Autodesk Inventor part; units mm, degrees
(part 5 of 6)
sketch "Sketch63" plane through (-95.5889, -143.7847, 10) normal (0, 0, -1) x (-0.7071068, 0.7071068, 0)
  line L0 (0, 6) -> (1.7, 6) projected
  line L1 (0, 6) -> (0, 0) projected
  line L2 (0, 0) -> (1.7, 0) projected
  line L3 (1.7, 6) -> (1.7, 0) projected
  line L4 (10.7, 0) -> (10.7, 6) projected
  line L5 (10.7, 0) -> (12.4, 0) projected
  line L6 (12.4, 0) -> (12.4, 6) projected
  line L7 (10.7, 6) -> (12.4, 6) projected
  line L8 (3.058, 5.3026) -> (4.2659, 6) projected
  line L9 (4.2659, 6) -> (1.7, 6) projected
  line L10 (1.7, 0) -> (1.7, 6) projected
  line L11 (1.7, 0) -> (6.0424, 0) projected
  line L12 (6.0424, 0) -> (3.058, 1.723) projected
  line L13 (3.058, 1.723) -> (3.058, 5.3026) projected
  line L14 (8.0501, 6) -> (9.258, 5.3026) projected
  line L15 (9.258, 5.3026) -> (9.258, 1.723) projected
  line L16 (9.258, 1.723) -> (6.2736, 0) projected
  line L17 (6.2736, 0) -> (10.7, 0) projected
  line L18 (10.7, 6) -> (10.7, 0) projected
  line L19 (10.7, 6) -> (8.0501, 6) projected
  line L20 (4.2659, 6) -> (8.0501, 6) projected
  circle A0 centre (6.158, 3.5128) radius 1.5 projected
  line L21 (4.2659, 6) -> (8.0501, 6) projected
  line L22 (3.058, 5.3026) -> (4.2659, 6) projected
  line L23 (3.058, 1.723) -> (3.058, 5.3026) projected
  line L24 (6.0424, 0) -> (3.058, 1.723) projected
  line L25 (6.2736, 0) -> (6.0424, 0) projected
  line L26 (9.258, 1.723) -> (6.2736, 0) projected
  line L27 (9.258, 5.3026) -> (9.258, 1.723) projected
  line L28 (8.0501, 6) -> (9.258, 5.3026) projected
  line L29 (-79.2698, 64.6815) -> (-78.0677, 63.4794) projected
  line L30 (-79.2698, 64.6815) -> (-83.5124, 60.4388) projected
  line L31 (-83.5124, 60.4388) -> (-82.3103, 59.2367) projected
  line L32 (-78.0677, 63.4794) -> (-82.3103, 59.2367) projected
  line L33 (-77.6457, 61.952) -> (-76.1357, 61.5474) projected
  line L34 (-76.1357, 61.5474) -> (-78.0677, 63.4794) projected
  line L35 (-82.3103, 59.2367) -> (-78.0677, 63.4794) projected
  line L36 (-82.3103, 59.2367) -> (-79.3285, 56.2549) projected
  line L37 (-79.3285, 56.2549) -> (-80.1768, 59.4208) projected
  line L38 (-80.1768, 59.4208) -> (-77.6457, 61.952) projected
  circle A1 centre (-76.7192, 58.4944) radius 1.5 projected
  circle A2 centre (-76.7192, 58.4944) radius 1.5 projected
  line L39 (-76.1357, 61.5474) -> (-73.6662, 59.0779) projected
  line L40 (-77.6457, 61.952) -> (-76.1357, 61.5474) projected
  line L41 (-80.1768, 59.4208) -> (-77.6457, 61.952) projected
  line L42 (-79.3285, 56.2549) -> (-80.1768, 59.4208) projected
  line L43 (-78.9587, 55.8851) -> (-79.3285, 56.2549) projected
  line L44 (-75.7928, 55.0368) -> (-78.9587, 55.8851) projected
  line L45 (-73.2616, 57.5679) -> (-75.7928, 55.0368) projected
  line L46 (-73.6662, 59.0779) -> (-73.2616, 57.5679) projected
  line L47 (-75.9464, 52.8728) -> (-71.7037, 57.1154) projected
  line L48 (-73.6662, 59.0779) -> (-73.2616, 57.5679) projected
  line L49 (-73.2616, 57.5679) -> (-75.7928, 55.0368) projected
  line L50 (-75.7928, 55.0368) -> (-78.9587, 55.8851) projected
  line L51 (-78.9587, 55.8851) -> (-75.9464, 52.8728) projected
  line L52 (-71.7037, 57.1154) -> (-75.9464, 52.8728) projected
  line L53 (-71.7037, 57.1154) -> (-73.6662, 59.0779) projected
  line L54 (-75.9464, 52.8728) -> (-71.7037, 57.1154) projected
  line L55 (-75.9464, 52.8728) -> (-74.7443, 51.6707) projected
  line L56 (-74.7443, 51.6707) -> (-70.5017, 55.9133) projected
  line L57 (-71.7037, 57.1154) -> (-70.5017, 55.9133) projected
  line L58 (-101.1831, 147.5831) -> (-106.1831, 147.5831) projected
  line L59 (-106.1831, 135.1831) -> (-106.1831, 147.5831) projected
  line L60 (-106.1831, 135.1831) -> (-101.1831, 135.1831) projected
  line L61 (-101.1831, 135.1831) -> (-101.1831, 147.5831) projected
  circle A3 centre (-103.7792, 141.4107) radius 1.5 projected
  line L62 (-129.1831, 145.8831) -> (-135.1831, 145.8831) projected
  line L63 (-129.1831, 147.5831) -> (-135.1831, 147.5831) projected
  line L64 (-133.569, 144.5107) -> (-129.9894, 144.5107) projected
  line L65 (-135.1831, 141.7149) -> (-133.569, 144.5107) projected
  line L66 (-133.569, 144.5107) -> (-129.9894, 144.5107) projected
  line L67 (-129.9894, 144.5107) -> (-129.1831, 143.1142) projected
  line L68 (-129.1831, 143.1142) -> (-129.1831, 145.8831) projected
  line L69 (-135.1831, 145.8831) -> (-129.1831, 145.8831) projected
  line L70 (-135.1831, 145.8831) -> (-135.1831, 141.7149) projected
  line L71 (-129.1831, 147.5831) -> (-129.1831, 145.8831) projected
  line L72 (-129.1831, 147.5831) -> (-135.1831, 147.5831) projected
  line L73 (-135.1831, 147.5831) -> (-135.1831, 145.8831) projected
  line L74 (-129.1831, 145.8831) -> (-135.1831, 145.8831) projected
  circle A4 centre (-131.7792, 141.4107) radius 1.5 projected
  line L75 (-135.1831, 141.1065) -> (-135.1831, 141.7149) projected
  line L76 (-133.569, 138.3107) -> (-135.1831, 141.1065) projected
  line L77 (-129.9894, 138.3107) -> (-133.569, 138.3107) projected
  line L78 (-129.1831, 139.7072) -> (-129.9894, 138.3107) projected
  line L79 (-129.1831, 143.1142) -> (-129.1831, 139.7072) projected
  line L80 (-129.9894, 144.5107) -> (-129.1831, 143.1142) projected
  line L81 (-133.569, 144.5107) -> (-129.9894, 144.5107) projected
  line L82 (-135.1831, 141.7149) -> (-133.569, 144.5107) projected
  line L83 (-133.569, 138.3107) -> (-135.1831, 141.1065) projected
  line L84 (-135.1831, 141.1065) -> (-135.1831, 136.8831) projected
  line L85 (-129.1831, 136.8831) -> (-135.1831, 136.8831) projected
  line L86 (-129.1831, 136.8831) -> (-129.1831, 139.7072) projected
  line L87 (-129.1831, 139.7072) -> (-129.9894, 138.3107) projected
  line L88 (-129.9894, 138.3107) -> (-133.569, 138.3107) projected
  line L89 (-135.1831, 135.1831) -> (-129.1831, 135.1831) projected
  line L90 (-135.1831, 136.8831) -> (-129.1831, 136.8831) projected
  line L91 (-135.1831, 136.8831) -> (-135.1831, 135.1831) projected
  line L92 (-135.1831, 135.1831) -> (-129.1831, 135.1831) projected
  line L93 (-129.1831, 136.8831) -> (-129.1831, 135.1831) projected
  line L94 (-79.6081, 145.9581) -> (-79.6081, 136.8081) projected
  line L95 (-86.1831, 145.9581) -> (-79.6081, 145.9581) projected
  line L96 (-86.1831, 136.8081) -> (-86.1831, 145.9581) projected
  line L97 (-86.1831, 136.8081) -> (-79.6081, 136.8081) projected
  line L98 (-86.1831, 145.9581) -> (-79.6081, 145.9581) projected
  line L99 (-79.6081, 145.9581) -> (-79.6081, 147.9581) projected
  line L100 (-79.6081, 147.9581) -> (-86.1831, 147.9581) projected
  line L101 (-86.1831, 147.9581) -> (-86.1831, 145.9581) projected
  line L102 (-86.1831, 136.8081) -> (-79.6081, 136.8081) projected
  line L103 (-86.1831, 136.8081) -> (-86.1831, 134.8081) projected
  line L104 (-86.1831, 134.8081) -> (-79.6081, 134.8081) projected
  line L105 (-79.6081, 134.8081) -> (-79.6081, 136.8081) projected
  line L106 (-43.4494, 188.6918) -> (-43.4494, 182.1168) projected
  line L107 (-43.4494, 188.6918) -> (-45.4494, 188.6918) projected
  line L108 (-45.4494, 188.6918) -> (-45.4494, 182.1168) projected
  line L109 (-45.4494, 182.1168) -> (-43.4494, 182.1168) projected
  line L110 (-34.2994, 182.1168) -> (-43.4494, 182.1168) projected
  line L111 (-34.2994, 188.6918) -> (-34.2994, 182.1168) projected
  line L112 (-43.4494, 188.6918) -> (-34.2994, 188.6918) projected
  line L113 (-43.4494, 188.6918) -> (-43.4494, 182.1168) projected
  line L114 (-34.2994, 188.6918) -> (-34.2994, 182.1168) projected
  line L115 (-34.2994, 182.1168) -> (-32.2994, 182.1168) projected
  line L116 (-32.2994, 182.1168) -> (-32.2994, 188.6918) projected
  line L117 (-32.2994, 188.6918) -> (-34.2994, 188.6918) projected
  circle A5 centre (-38.9335, 206.21) radius 1.5 projected
  line L118 (-32.6744, 203.6918) -> (-32.6744, 208.6918) projected
  line L119 (-45.0744, 208.6918) -> (-32.6744, 208.6918) projected
  line L120 (-45.0744, 208.6918) -> (-45.0744, 203.6918) projected
  line L121 (-45.0744, 203.6918) -> (-32.6744, 203.6918) projected
  line L122 (-35.8335, 232.4202) -> (-37.0951, 231.6918) projected
  line L123 (-37.0951, 231.6918) -> (-34.3744, 231.6918) projected
  line L124 (-34.3744, 237.6918) -> (-34.3744, 231.6918) projected
  line L125 (-34.3744, 237.6918) -> (-38.7642, 237.6918) projected
  line L126 (-38.7642, 237.6918) -> (-35.8335, 235.9998) projected
  line L127 (-35.8335, 235.9998) -> (-35.8335, 232.4202) projected
  line L128 (-32.6744, 231.6918) -> (-34.3744, 231.6918) projected
  line L129 (-32.6744, 231.6918) -> (-32.6744, 237.6918) projected
  line L130 (-32.6744, 237.6918) -> (-34.3744, 237.6918) projected
  line L131 (-34.3744, 231.6918) -> (-34.3744, 237.6918) projected
  circle A6 centre (-38.9335, 234.21) radius 1.5 projected
  line L132 (-37.0951, 231.6918) -> (-40.7719, 231.6918) projected
  line L133 (-35.8335, 232.4202) -> (-37.0951, 231.6918) projected
  line L134 (-35.8335, 235.9998) -> (-35.8335, 232.4202) projected
  line L135 (-38.7642, 237.6918) -> (-35.8335, 235.9998) projected
  line L136 (-39.1028, 237.6918) -> (-38.7642, 237.6918) projected
  line L137 (-42.0335, 235.9998) -> (-39.1028, 237.6918) projected
  line L138 (-42.0335, 232.4202) -> (-42.0335, 235.9998) projected
  line L139 (-40.7719, 231.6918) -> (-42.0335, 232.4202) projected
  line L140 (-42.0335, 235.9998) -> (-39.1028, 237.6918) projected
  line L141 (-43.3744, 237.6918) -> (-43.3744, 231.6918) projected
  line L142 (-43.3744, 237.6918) -> (-43.3744, 231.6918) projected
  line L143 (-43.3744, 237.6918) -> (-45.0744, 237.6918) projected
  line L144 (-45.0744, 237.6918) -> (-45.0744, 231.6918) projected
  line L145 (-43.3744, 231.6918) -> (-45.0744, 231.6918) projected
  line L146 (-40.7719, 231.6918) -> (-42.0335, 232.4202) projected
  line L147 (-42.0335, 232.4202) -> (-42.0335, 235.9998) projected
  line L148 (-42.0335, 235.9998) -> (-39.1028, 237.6918) projected
  line L149 (-39.1028, 237.6918) -> (-43.3744, 237.6918) projected
  line L150 (-43.3744, 231.6918) -> (-43.3744, 237.6918) projected
  line L151 (-43.3744, 231.6918) -> (-40.7719, 231.6918) projected
  line L152 (3.9214, 145.5746) -> (8.5707, 150.2238) projected
  line L153 (3.9214, 145.5746) -> (8.5707, 150.2238) projected
  line L154 (8.5707, 150.2238) -> (7.1565, 151.638) projected
  line L155 (7.1565, 151.638) -> (2.5072, 146.9888) projected
  line L156 (2.5072, 146.9888) -> (3.9214, 145.5746) projected
  line L157 (10.3915, 139.1046) -> (3.9214, 145.5746) projected
  line L158 (10.3915, 139.1046) -> (15.0407, 143.7538) projected
  line L159 (8.5707, 150.2238) -> (15.0407, 143.7538) projected
  line L160 (3.9214, 145.5746) -> (8.5707, 150.2238) projected
  line L161 (10.3915, 139.1046) -> (15.0407, 143.7538) projected
  line L162 (10.3915, 139.1046) -> (11.8057, 137.6904) projected
  line L163 (11.8057, 137.6904) -> (16.4549, 142.3396) projected
  line L164 (16.4549, 142.3396) -> (15.0407, 143.7538) projected
  line L165 (26.7963, 153.2113) -> (30.3319, 156.7469) projected
  line L166 (21.5638, 165.515) -> (30.3319, 156.7469) projected
  line L167 (21.5638, 165.515) -> (18.0282, 161.9795) projected
  line L168 (18.0282, 161.9795) -> (26.7963, 153.2113) projected
  circle A7 centre (24.1798, 159.3656) radius 1.5 projected
  line L169 (43.2719, 184.819) -> (39.0293, 180.5764) projected
  line L170 (43.2719, 184.819) -> (42.0699, 186.0211) projected
  line L171 (42.0699, 186.0211) -> (37.8272, 181.7785) projected
  line L172 (39.0293, 180.5764) -> (37.8272, 181.7785) projected
  line L173 (40.8896, 178.7161) -> (40.5212, 180.0911) projected
  line L174 (40.5212, 180.0911) -> (43.0523, 182.6222) projected
  line L175 (43.0523, 182.6222) -> (46.3532, 181.7377) projected
  line L176 (46.3532, 181.7377) -> (43.2719, 184.819) projected
  line L177 (39.0293, 180.5764) -> (43.2719, 184.819) projected
  line L178 (39.0293, 180.5764) -> (40.8896, 178.7161) projected
  circle A8 centre (43.9788, 179.1646) radius 1.5 projected
  line L179 (43.5302, 176.0754) -> (40.8896, 178.7161) projected
  line L180 (44.9052, 175.707) -> (43.5302, 176.0754) projected
  line L181 (47.4364, 178.2381) -> (44.9052, 175.707) projected
  line L182 (46.5519, 181.5391) -> (47.4364, 178.2381) projected
  line L183 (46.3532, 181.7377) -> (46.5519, 181.5391) projected
  line L184 (43.0523, 182.6222) -> (46.3532, 181.7377) projected
  line L185 (40.5212, 180.0911) -> (43.0523, 182.6222) projected
  line L186 (40.8896, 178.7161) -> (40.5212, 180.0911) projected
  line L187 (44.9052, 175.707) -> (43.5302, 176.0754) projected
  line L188 (43.5302, 176.0754) -> (45.3933, 174.2124) projected
  line L189 (49.6359, 178.4551) -> (45.3933, 174.2124) projected
  line L190 (49.6359, 178.4551) -> (46.5519, 181.5391) projected
  line L191 (46.5519, 181.5391) -> (47.4364, 178.2381) projected
  line L192 (47.4364, 178.2381) -> (44.9052, 175.707) projected
  line L193 (46.5953, 173.0103) -> (45.3933, 174.2124) projected
  line L194 (46.5953, 173.0103) -> (50.838, 177.253) projected
  line L195 (50.838, 177.253) -> (49.6359, 178.4551) projected
  line L196 (45.3933, 174.2124) -> (49.6359, 178.4551) projected
  line L197 (46.9337, 91.7337) -> (46.9337, 100.8837) projected
  line L198 (53.5087, 91.7337) -> (46.9337, 91.7337) projected
  line L199 (53.5087, 100.8837) -> (53.5087, 91.7337) projected
  line L200 (53.5087, 100.8837) -> (46.9337, 100.8837) projected
  line L201 (53.5087, 100.8837) -> (46.9337, 100.8837) projected
  line L202 (53.5087, 100.8837) -> (53.5087, 102.8837) projected
  line L203 (53.5087, 102.8837) -> (46.9337, 102.8837) projected
  line L204 (46.9337, 102.8837) -> (46.9337, 100.8837) projected
  line L205 (53.5087, 91.7337) -> (46.9337, 91.7337) projected
  line L206 (46.9337, 91.7337) -> (46.9337, 89.7337) projected
  line L207 (46.9337, 89.7337) -> (53.5087, 89.7337) projected
  line L208 (53.5087, 89.7337) -> (53.5087, 91.7337) projected
  circle A9 centre (71.0354, 96.2907) radius 1.5 projected
  line L209 (68.5087, 90.1087) -> (73.5087, 90.1087) projected
  line L210 (73.5087, 102.5087) -> (73.5087, 90.1087) projected
  line L211 (73.5087, 102.5087) -> (68.5087, 102.5087) projected
  line L212 (68.5087, 102.5087) -> (68.5087, 90.1087) projected
  line L213 (102.5087, 100.8087) -> (96.5087, 100.8087) projected
  line L214 (102.5087, 100.8087) -> (102.5087, 102.5087) projected
  line L215 (102.5087, 102.5087) -> (96.5087, 102.5087) projected
  line L216 (96.5087, 100.8087) -> (96.5087, 102.5087) projected
  line L217 (100.8251, 99.3907) -> (102.5087, 96.4747) projected
  line L218 (102.5087, 96.4747) -> (102.5087, 100.8087) projected
  line L219 (96.5087, 100.8087) -> (102.5087, 100.8087) projected
  line L220 (96.5087, 100.8087) -> (96.5087, 98.1143) projected
  line L221 (96.5087, 98.1143) -> (97.2456, 99.3907) projected
  line L222 (97.2456, 99.3907) -> (100.8251, 99.3907) projected
  circle A10 centre (99.0354, 96.2907) radius 1.5 projected
  line L223 (102.5087, 96.4747) -> (102.5087, 96.1066) projected
  line L224 (100.8251, 99.3907) -> (102.5087, 96.4747) projected
  line L225 (97.2456, 99.3907) -> (100.8251, 99.3907) projected
  line L226 (96.5087, 98.1143) -> (97.2456, 99.3907) projected
  line L227 (96.5087, 94.467) -> (96.5087, 98.1143) projected
  line L228 (97.2456, 93.1907) -> (96.5087, 94.467) projected
  line L229 (100.8251, 93.1907) -> (97.2456, 93.1907) projected
  line L230 (102.5087, 96.1066) -> (100.8251, 93.1907) projected
  line L231 (102.5087, 96.1066) -> (100.8251, 93.1907) projected
  line L232 (100.8251, 93.1907) -> (97.2456, 93.1907) projected
  line L233 (97.2456, 93.1907) -> (96.5087, 94.467) projected
  line L234 (96.5087, 94.467) -> (96.5087, 91.8087) projected
  line L235 (102.5087, 91.8087) -> (96.5087, 91.8087) projected
  line L236 (102.5087, 91.8087) -> (102.5087, 96.1066) projected
  line L237 (96.5087, 90.1087) -> (96.5087, 91.8087) projected
  line L238 (96.5087, 90.1087) -> (102.5087, 90.1087) projected
  line L239 (102.5087, 90.1087) -> (102.5087, 91.8087) projected
  line L240 (96.5087, 91.8087) -> (102.5087, 91.8087) projected
  circle A11 centre (6.158, 31.5128) radius 1.5 projected
  line L241 (0, 34) -> (0, 29) projected
  line L242 (12.4, 29) -> (0, 29) projected
  line L243 (12.4, 29) -> (12.4, 34) projected
  line L244 (12.4, 34) -> (0, 34) projected
  line L245 (1.625, 55.575) -> (10.775, 55.575) projected
  line L246 (1.625, 49) -> (1.625, 55.575) projected
  line L247 (10.775, 49) -> (1.625, 49) projected
  line L248 (10.775, 49) -> (10.775, 55.575) projected
  line L249 (1.625, 49) -> (1.625, 55.575) projected
  line L250 (1.625, 55.575) -> (-0.375, 55.575) projected
  line L251 (-0.375, 55.575) -> (-0.375, 49) projected
  line L252 (-0.375, 49) -> (1.625, 49) projected
  line L253 (10.775, 49) -> (10.775, 55.575) projected
  line L254 (10.775, 49) -> (12.775, 49) projected
  line L255 (12.775, 49) -> (12.775, 55.575) projected
  line L256 (12.775, 55.575) -> (10.775, 55.575) projected
  line L257 (-47.7151, 93.938) -> (-43.0659, 98.5872) projected
  line L258 (-43.0659, 98.5872) -> (-44.4801, 100.0015) projected
  line L259 (-44.4801, 100.0015) -> (-49.1294, 95.3522) projected
  line L260 (-49.1294, 95.3522) -> (-47.7151, 93.938) projected
  line L261 (-43.0659, 98.5872) -> (-36.5959, 92.1172) projected
  line L262 (-47.7151, 93.938) -> (-43.0659, 98.5872) projected
  line L263 (-41.2451, 87.468) -> (-47.7151, 93.938) projected
  line L264 (-41.2451, 87.468) -> (-36.5959, 92.1172) projected
  line L265 (-41.2451, 87.468) -> (-36.5959, 92.1172) projected
  line L266 (-41.2451, 87.468) -> (-39.8309, 86.0538) projected
  line L267 (-39.8309, 86.0538) -> (-35.1817, 90.703) projected
  line L268 (-35.1817, 90.703) -> (-36.5959, 92.1172) projected
  line L269 (-59.4708, 84.4805) -> (-63.0063, 80.9449) projected
  line L270 (-54.2382, 72.1768) -> (-63.0063, 80.9449) projected
  line L271 (-54.2382, 72.1768) -> (-50.7027, 75.7123) projected
  line L272 (-50.7027, 75.7123) -> (-59.4708, 84.4805) projected
  circle A12 centre (-56.9202, 78.2934) radius 1.5 projected
  point P0 (34.0795, 169.2627)
  point P1 (-75.9464, 52.8728)
  point P2 (-71.7037, 57.1154)
  point P3 (-73.6662, 59.0779)
  point P4 (-76.1357, 61.5474)
  point P5 (-78.0677, 63.4794)
  point P6 (96.5087, 94.467)
  point P7 (96.5087, 91.8087)
  point P8 (102.5087, 91.8087)
  point P9 (102.5087, 96.1066)
  point P10 (102.5087, 96.4747)
  point P11 (46.9337, 100.8837)
  point P12 (46.9337, 91.7337)
  point P13 (53.5087, 91.7337)
  point P14 (53.5087, 100.8837)
  point P15 (15.0407, 143.7538)
  point P16 (8.5707, 150.2238)
  point P17 (3.9214, 145.5746)
  point P18 (10.3915, 139.1046)
  point P19 (46.3532, 181.7377)
  point P20 (43.2719, 184.819)
  point P21 (39.0293, 180.5764)
  point P22 (40.8896, 178.7161)
  point P23 (43.5302, 176.0754)
  point P24 (45.3933, 174.2124)
  point P25 (49.6359, 178.4551)
  point P26 (46.5519, 181.5391)
  point P27 (-43.4494, 182.1168)
  point P28 (-34.2994, 182.1168)
  point P29 (-34.2994, 188.6918)
  point P30 (-43.4494, 188.6918)
  point P31 (-43.3744, 237.6918)
  point P32 (-40.7719, 231.6918)
  point P33 (-37.0951, 231.6918)
  point P34 (-34.3744, 231.6918)
  point P35 (-34.3744, 237.6918)
  point P36 (-38.7642, 237.6918)
  point P37 (-39.1028, 237.6918)
  point P38 (-135.1831, 145.8831)
  point P39 (-135.1831, 141.7149)
  point P40 (-135.1831, 141.1065)
  point P41 (-129.1831, 143.1142)
  point P42 (-129.1831, 145.8831)
  point P43 (-129.1831, 147.5831)
  point P44 (-79.6081, 136.8081)
  point P45 (-79.6081, 145.9581)
  point P46 (-86.1831, 145.9581)
  point P47 (-86.1831, 136.8081)
  point P48 (-47.7151, 93.938)
  point P49 (-41.2451, 87.468)
  point P50 (-43.0659, 98.5872)
  point P51 (1.625, 49)
  point P52 (10.775, 49)
  point P53 (10.775, 55.575)
  point P54 (1.625, 55.575)
  point P55 (10.7, 6)
  point P56 (1.7, 0)
  point P57 (6.0424, 0)
  point P58 (6.2736, 0)
  point P59 (10.7, 0)
extrude "Extrusion60" cut sketch "Sketch63" against normal blind 19 contours L0 L3 L2 L1 | L9 L8 L13 L12 L11 L3 | L20 L14 L15 L16 L25 L12 L13 L8 | L19 L4 L17 L16 L15 L14 | L7 L6 L5 L4 | L29 L32 L31 L30 | L34 L33 L38 L37 L36 L32 | L39 L46 L45 L44 L43 L37 L38 L33 | L53 L47 L51 L44 L45 L46 | L57 L56 L55 L47 | A1 | L61 L60 L59 L58 | L68 L67 L64 L65 L70 L62 | L62 L73 L63 L71 | L79 L78 L77 L76 L75 L65 L64 L67 | L86 L85 L84 L76 L77 L78 | L93 L89 L91 L85 | A4 | L94 L97 L96 L95 | L95 L101 L100 L99 | L105 L104 L103 L97 | L112 L111 L110 L106 | L106 L109 L108 L107 | L117 L116 L115 L111 | L121 L120 L119 L118 | L127 L126 L125 L124 L123 L122 | L122 L132 L139 L138 L137 L136 L126 L127 | L124 L130 L129 L128 | L151 L141 L149 L137 L138 L139 | L145 L144 L143 L141 | L156 L155 L154 L152 | L152 L159 L158 L157 | L158 L164 L163 L162 | L168 L167 L166 L165 | L176 L175 L174 L173 L178 L169 | L169 L172 L171 L170 | L183 L182 L181 L180 L179 L173 L174 L175 | L190 L189 L188 L180 L181 L182 | L195 L194 L193 L189 | A8 | L197 L200 L199 L198 | L198 L208 L207 L206 | L204 L203 L202 L200 | A9 | L212 L211 L210 L209 | L218 L217 L222 L221 L220 L213 | L213 L216 L215 L214 | L223 L230 L229 L228 L227 L221 L222 L217 | L236 L235 L234 L228 L229 L230 | L239 L238 L237 L235 | A10 | L244 L243 L242 L241 | L245 L248 L247 L246 | L246 L252 L251 L250 | L256 L255 L254 L248 | L260 L259 L258 L257 | L257 L261 L264 L263 | L264 L268 L267 L266 | L272 L271 L270 L269
sketch "Sketch66" plane through (9.4148, -138.9501, 55) normal (0, 0, -1) x (-1, 0, 0)
  line L0 (-45.5215, 41.2849) -> (-35.0215, 41.2849)
  line L1 (-31.4215, 41.2849) -> (-20.9215, 41.2849)
  line L2 (-17.3215, 41.2849) -> (-6.8215, 41.2849)
  line L3 (-3.2285, 41.2849) -> (31.7715, 41.2849)
  line L4 (-74.8673, 64.1) -> (-74.8673, 71.1) projected
  line L5 (77.0633, 52.65) -> (77.0633, 82.65) projected
  arc A0 (-40.1627, 65.6758) -> (-45.5215, 41.2849) centre (7.9948, 42.3113) ccw
  arc A1 (-28.0472, 65.6798) -> (-35.0215, 41.2849) centre (4.8127, 43.091) ccw
  arc A2 (-23.5743, 65.6813) -> (-31.4215, 41.2849) centre (4.8107, 43.0909) ccw
  arc A3 (-7.8955, 65.6864) -> (-20.9215, 41.2849) centre (5.751, 42.7242) ccw
  arc A4 (2.9932, 65.69) -> (-17.3215, 41.2849) centre (5.416, 43.0158) ccw
  arc A5 (4.8107, 55.3031) -> (-6.8215, 41.2849) centre (5.3934, 42.9843) ccw
  arc A6 (4.8107, 51.7737) -> (-3.2285, 41.2849) centre (5.7806, 42.7051) ccw
  arc A7 (-39.2025, 67.5594) -> (-40.1627, 65.6758) centre (7.9948, 42.3113) ccw
  arc A8 (-45.5215, 94.0365) -> (-39.2025, 67.5594) centre (6.2562, 92.4012) ccw
  line L6 (-45.5215, 94.0365) -> (-35.0215, 94.0365)
  line L7 (-31.4215, 94.0365) -> (-20.9215, 94.0365)
  line L8 (-17.3215, 94.0365) -> (-6.8215, 94.0365)
  line L9 (-3.2215, 94.0365) -> (31.7785, 94.0365)
  arc A9 (31.7715, 41.2849) -> (31.7785, 94.0365) centre (30.1154, 67.6609) ccw
  arc A10 (-26.5935, 67.6609) -> (-28.0472, 65.6798) centre (4.8127, 43.091) ccw
  arc A11 (-35.0215, 94.0365) -> (-26.5935, 67.6609) centre (5.544, 92.4644) ccw
  arc A12 (-21.8792, 67.6609) -> (-23.5743, 65.6813) centre (4.8107, 43.0909) ccw
  arc A13 (-31.4215, 94.0365) -> (-21.8792, 67.6609) centre (3.6645, 91.8162) ccw
  arc A14 (-4.0829, 67.5594) -> (-7.8955, 65.6864) centre (5.751, 42.7242) ccw
  arc A15 (-20.9215, 94.0365) -> (-4.0829, 67.5594) centre (5.8906, 92.4952) ccw
  line L10 (4.8107, 51.7737) -> (30.8107, 51.7737)
  line L11 (4.8107, 55.3031) -> (30.8107, 55.3031)
  line L12 (4.8107, 79.8559) -> (30.8107, 79.8559)
  arc A16 (-6.8215, 94.0365) -> (4.8107, 79.8559) centre (5.796, 92.5253) ccw
  arc A17 (30.8107, 55.3031) -> (42.559, 65.703) centre (29.9904, 68.0655) ccw
  line L13 (2.9932, 65.69) -> (42.559, 65.703)
  line L14 (2.9932, 69.2913) -> (42.5593, 69.2913)
  arc A18 (42.5593, 69.2913) -> (30.8107, 79.8559) centre (29.7982, 66.9149) ccw
  arc A19 (-17.3215, 94.0365) -> (2.9932, 69.2913) centre (6.0846, 92.5405) ccw
  line L15 (30.8622, 83.4409) -> (4.8622, 83.4409)
  arc A20 (-3.2215, 94.0365) -> (4.8622, 83.4409) centre (6.2101, 92.8507) ccw
  arc A21 (30.8107, 51.7737) -> (30.8622, 83.4409) centre (30.389, 67.608) ccw
  line L16 (-30.6501, 104.1104) -> (-26.9242, 104.1104) projected
  line L17 (-26.9242, 31.1897) -> (-30.6501, 31.1897) projected
  line L18 (0, 0) -> (18.8297, 0) projected
  line L19 (0, 135.3001) -> (0, 134.0127) projected
  point P0 (9.4148, 138.9501)
  point P1 (-23.5743, 65.6813)
  dimension "d833" = 10.5
  dimension "d834" = 10.5
  dimension "d835" = 3.6
  dimension "d836" = 10.5
  dimension "d837" = 3.6
  dimension "d838" = 35
  dimension "d839" = 3.593
  dimension "d842" = 10.5
  dimension "d843" = 10.5
  dimension "d844" = 3.6
  dimension "d845" = 10.5
  dimension "d846" = 3.6
  dimension "d847" = 35
  dimension "d848" = 3.6
  dimension "d849" = 26
  dimension "d850" = 26
  dimension "d851" = 26
  dimension "d882" = 34.504
  dimension "d883" = 34.5043
  dimension "d884" = 45.2848
  dimension "d886" = 46.2526
  dimension "d896" = 72.2506
  dimension "d900" = 81.1462
  dimension "d901" = 98.9425
  dimension "d902" = 26
  dimension "d905" = 14.1496
  dimension "d911" = 10.0952
  dimension "d912" = 10.0739
  dimension "d913" = 15.8399
  dimension "d914" = 26.428
  dimension "d915" = 12.7888
  dimension "d916" = 12.9805
  dimension "d917" = 53.5261
  dimension "d918" = 51.8036
  dimension "d919" = 9.5059
  dimension "d920" = 23.4538
  dimension "d921" = 26.8564
  dimension "d922" = 12.7077
  dimension "d923" = 9.1203
  dimension "d924" = 26.7113
  dimension "d925" = 26.7113
  dimension "d926" = 40.5959
  dimension "d927" = 22.8033
  dimension "d928" = 12.3325
  dimension "d929" = 39.8752
  dimension "d930" = 39.8752
  dimension "d931" = 36.2772
  dimension "d932" = 36.2772
  dimension "d933" = 35.1562
  dimension "d934" = 89.981
  dimension "d935" = 69.2913
  dimension "d936" = 55.303
  dimension "d937" = 51.7737
  dimension "d938" = 79.8559
  dimension "d939" = 41.2849
  dimension "d940" = 94.0365
  dimension "d941" = 41.2849
  dimension "d942" = 94.0365
  dimension "d943" = 41.2849
  dimension "d944" = 16.9356
  dimension "d945" = 45.2918
  dimension "d946" = 46.2011
  dimension "d947" = 69.0685
  dimension "d948" = 70.8071
  constraints: 46 point on circle, 28 end point, 22 centre point, 13 horizontal, 2 vertical alignment, 1 concentric, 1 point on line
  measures "d833" distance of L0.start L0.end
  measures "d834" distance of L1.start L1.end
  measures "d835" distance of L1.start L0.end
  measures "d836" distance of L2.start L2.end
  measures "d837" distance of L2.start L1.end
  measures "d838" distance of L3.start L3.end
  measures "d839" distance of L3.start L2.end
  measures "d842" distance of L6.start L6.end
  measures "d843" distance of L7.start L7.end
  measures "d844" distance of L7.start L6.end
  measures "d845" distance of L8.start L8.end
  measures "d846" distance of L8.start L7.end
  measures "d847" distance of L9.start L9.end
  measures "d848" distance of L9.start L8.end
  measures "d849" distance of L10.start L10.end
  measures "d850" distance of L11.start L11.end
  measures "d851" distance of L12.start L12.end
  measures "d882" distance from line of L14.end L5
  measures "d883" distance from line of L13.end L5
  measures "d884" distance from line of L9.end L5
  measures "d886" distance from line of L12.end L5
  measures "d896" distance from line of A10.centre L5
  measures "d900" distance from line of A14.start L5
  measures "d901" distance from line of A12.start L5
  measures "d902" distance of L15.start L15.end
  measures "d905" distance between parallel lines of L15 L14
  measures "d911" distance between parallel lines of L1 L17
  measures "d912" distance between parallel lines of L16 L7
  measures "d913" radius of A21
  measures "d914" radius of A9
  measures "d915" radius of A17
  measures "d916" radius of A18
  measures "d917" radius of A0
  measures "d918" radius of A8
  measures "d919" radius of A20
  measures "d920" radius of A19
  measures "d921" radius of A15
  measures "d922" radius of A16
  measures "d923" radius of A6
  measures "d924" radius of A3
  measures "d925" radius of A14
  measures "d926" radius of A11
  measures "d927" radius of A4
  measures "d928" radius of A5
  measures "d929" radius of A1
  measures "d930" radius of A10
  measures "d931" radius of A2
  measures "d932" radius of A12
  measures "d933" radius of A13
  measures "d934" angle of L19 L13
  measures "d935" distance between parallel lines of L18 L14
  measures "d936" distance between parallel lines of L18 L11
  measures "d937" distance between parallel lines of L18 L10
  measures "d938" distance between parallel lines of L18 L12
  measures "d939" distance between parallel lines of L18 L3
  measures "d940" distance between parallel lines of L18 L9
  measures "d941" distance between parallel lines of L18 L2
  measures "d942" distance between parallel lines of L18 L6
  measures "d943" distance between parallel lines of L18 L0
  measures "d944" distance from line of L5.end L13
  measures "d945" distance from line of L3.end L5
  measures "d946" distance from line of L15.start L5
  measures "d947" distance from line of A0.centre L5
  measures "d948" distance from line of A8.centre L5
extrude "Extrusion61" cut sketch "Sketch66" against normal blind 92.5
sketch "Sketch67" plane through (88.2822, -48.8001, 10) normal (1, 0, 0) x (0, 0, -1)
  line L0 (0, -22.5) -> (-58.1963, -22.5) projected
  line L1 (0, -45) -> (0, 0) projected
  line L2 (-56.7845, 0) -> (0, 0) projected
  line L3 (0, -45) -> (-56.7845, -45) projected
  line L4 (-6.15, -26.05) -> (-6.15, -19.05) projected
  arc A0 (-2.35, -19.05) -> (-6.15, -19.05) centre (-4.25, -19.05) ccw projected
  line L5 (-2.35, -19.05) -> (-2.35, -26.05) projected
  arc A1 (-6.15, -26.05) -> (-2.35, -26.05) centre (-4.25, -26.05) ccw projected
  circle A2 centre (-3.5, -1.55) radius 1 projected
  circle A3 centre (-12, -9.05) radius 8.15 projected
  circle A4 centre (-20.5, -1.55) radius 1 projected
  circle A5 centre (-20.5, -43.55) radius 1 projected
  circle A6 centre (-12, -36.05) radius 8.15 projected
  circle A7 centre (-3.5, -43.55) radius 1 projected
  line L6 (0, -45) -> (-25, -45)
  line L7 (-25, -45) -> (-25, 0)
  line L8 (-25, 0) -> (0, 0)
  line L9 (0, 0) -> (0, -45)
  arc A8 (-56.7845, 0) -> (-56.7845, -45) centre (121.8037, -22.5) ccw projected
  point P0 (10, 48.8001)
  dimension "d966" = 25
  constraints: 8 end point, 2 parallel, 1 horizontal, 1 perpendicular, 1 point on line
  measures "d966" distance of L7.end L8.end
extrude "Extrusion62" cut sketch "Sketch67" against normal blind 10 contours L1 L3 L7 L0 L4 A1 L5 | L0 L5 A0 L4 L7 L2 L1 | L5 A1 L4 L0 | L0 L4 A0 L5 | A2 | A3 | A4 | A5 | A6 | A7
sketch "Sketch71" plane through (9.4148, -138.9501, 55) normal (0, 0, -1) x (-1, 0, 0)
  line L0 (2.9932, 65.69) -> (42.559, 65.703) projected
  arc A0 (30.8107, 55.3031) -> (42.559, 65.703) centre (29.9904, 68.0655) ccw projected
  line L1 (30.8107, 55.3031) -> (4.8107, 55.3031) projected
  arc A1 (4.8107, 55.3031) -> (-6.8215, 41.2849) centre (5.3934, 42.9843) ccw projected
  line L2 (-6.8215, 41.2849) -> (-17.3215, 41.2849) projected
  arc A2 (2.9932, 65.69) -> (-17.3215, 41.2849) centre (5.416, 43.0158) ccw projected
  arc A3 (-20.9215, 94.0365) -> (-4.0829, 67.5594) centre (5.8906, 92.4952) ccw projected
  arc A4 (-4.0829, 67.5594) -> (-20.9215, 41.2849) centre (5.751, 42.7242) ccw projected
  line L3 (-20.9215, 41.2849) -> (-31.4215, 41.2849) projected
  arc A5 (-21.8792, 67.6609) -> (-31.4215, 41.2849) centre (4.8107, 43.0909) ccw projected
  arc A6 (-31.4215, 94.0365) -> (-21.8792, 67.6609) centre (3.6645, 91.8162) ccw projected
  line L4 (-31.4215, 94.0365) -> (-20.9215, 94.0365) projected
  arc A7 (30.8107, 51.7737) -> (30.8622, 83.4409) centre (30.389, 67.608) ccw projected
  line L5 (30.8622, 83.4409) -> (4.8622, 83.4409) projected
  arc A8 (-3.2215, 94.0365) -> (4.8622, 83.4409) centre (6.2101, 92.8507) ccw projected
  line L6 (-3.2215, 94.0365) -> (31.7785, 94.0365) projected
  arc A9 (31.7715, 41.2849) -> (31.7785, 94.0365) centre (30.1154, 67.6609) ccw projected
  line L7 (31.7715, 41.2849) -> (-3.2285, 41.2849) projected
  arc A10 (4.8107, 51.7737) -> (-3.2285, 41.2849) centre (5.7806, 42.7051) ccw projected
  line L8 (4.8107, 51.7737) -> (30.8107, 51.7737) projected
  line L9 (-45.5215, 94.0365) -> (-35.0215, 94.0365) projected
  arc A11 (-35.0215, 94.0365) -> (-26.5935, 67.6609) centre (5.544, 92.4644) ccw projected
  arc A12 (-26.5935, 67.6609) -> (-35.0215, 41.2849) centre (4.8127, 43.091) ccw projected
  line L10 (-35.0215, 41.2849) -> (-45.5215, 41.2849) projected
  arc A13 (-39.2025, 67.5594) -> (-45.5215, 41.2849) centre (7.9948, 42.3113) ccw projected
  arc A14 (-45.5215, 94.0365) -> (-39.2025, 67.5594) centre (6.2562, 92.4012) ccw projected
  arc A15 (-6.8215, 94.0365) -> (4.8107, 79.8559) centre (5.796, 92.5253) ccw projected
  line L11 (4.8107, 79.8559) -> (30.8107, 79.8559) projected
  arc A16 (42.5593, 69.2913) -> (30.8107, 79.8559) centre (29.7982, 66.9149) ccw projected
  line L12 (42.5593, 69.2913) -> (2.9932, 69.2913) projected
  arc A17 (-17.3215, 94.0365) -> (2.9932, 69.2913) centre (6.0846, 92.5405) ccw projected
  line L13 (-17.3215, 94.0365) -> (-6.8215, 94.0365) projected
  line L14 (-82.4666, 113.9315) -> (-81.0911, 112.5559) projected
  line L15 (-81.0911, 112.5559) -> (-77.2122, 98.9398) projected
  line L16 (-77.2122, 98.9398) -> (-69.5183, 101.1316) projected
  line L17 (-69.5183, 101.1316) -> (-67.3265, 93.4378) projected
  line L18 (-67.3265, 93.4378) -> (-75.0204, 91.2459) projected
  line L19 (-75.0204, 91.2459) -> (-74.8673, 90.15) projected
  line L20 (-74.8673, 90.15) -> (-74.8673, 45.15) projected
  line L21 (-74.8673, 45.15) -> (-75.0204, 44.0541) projected
  line L22 (-75.0204, 44.0541) -> (-67.3265, 41.8623) projected
  line L23 (-67.3265, 41.8623) -> (-69.5183, 34.1684) projected
  line L24 (-69.5183, 34.1684) -> (-77.2122, 36.3602) projected
  line L25 (-77.2122, 36.3602) -> (-81.0911, 22.7441) projected
  line L26 (-81.0911, 22.7441) -> (-82.4666, 21.3686) projected
  line L27 (-69.0444, 7.9464) -> (-68.5062, 8.4845) projected
  line L28 (-68.5062, 8.4845) -> (-50.0258, 20.9649) projected
  line L29 (-50.0258, 20.9649) -> (-49.6501, 21.1897) projected
  line L30 (-49.6501, 21.1897) -> (-30.6501, 31.1897) projected
  line L31 (-30.6501, 31.1897) -> (-26.9242, 31.1897) projected
  line L32 (-26.9242, 31.1897) -> (-7.9242, 21.1897) projected
  line L33 (-7.9242, 21.1897) -> (-6, 18.9375) projected
  line L34 (-6, 18.9375) -> (0, 1.2874) projected
  line L35 (0, 1.2874) -> (0, 0) projected
  line L36 (0, 0) -> (18.8297, 0) projected
  line L37 (18.8297, 0) -> (18.8297, 1.2874) projected
  line L38 (18.8297, 1.2874) -> (24.8297, 18.9375) projected
  line L39 (24.8297, 18.9375) -> (26.7539, 21.1897) projected
  line L40 (26.7539, 21.1897) -> (45.7539, 31.1897) projected
  line L41 (45.7539, 31.1897) -> (49.4798, 31.1897) projected
  line L42 (49.4798, 31.1897) -> (68.4798, 21.1897) projected
  line L43 (68.4798, 21.1897) -> (68.8555, 20.9649) projected
  line L44 (68.8555, 20.9649) -> (87.3359, 8.4845) projected
  line L45 (101.1576, 21.2299) -> (100.068, 22.3196) projected
  line L46 (100.068, 22.3196) -> (87.603, 52.65) projected
  line L47 (87.603, 52.65) -> (77.0633, 52.65) projected
  line L48 (77.0633, 52.65) -> (77.0633, 82.65) projected
  line L49 (77.0633, 82.65) -> (87.603, 82.65) projected
  line L50 (87.603, 82.65) -> (100.068, 112.9805) projected
  line L51 (100.068, 112.9805) -> (101.1576, 114.0701) projected
  line L52 (87.874, 127.3537) -> (87.3359, 126.8156) projected
  line L53 (87.3359, 126.8156) -> (68.8555, 114.3352) projected
  line L54 (68.8555, 114.3352) -> (68.4798, 114.1104) projected
  line L55 (68.4798, 114.1104) -> (49.4798, 104.1104) projected
  line L56 (49.4798, 104.1104) -> (45.7539, 104.1104) projected
  line L57 (45.7539, 104.1104) -> (26.7539, 114.1104) projected
  line L58 (26.7539, 114.1104) -> (24.8297, 116.3626) projected
  line L59 (24.8297, 116.3626) -> (18.8297, 134.0127) projected
  line L60 (18.8297, 134.0127) -> (18.8297, 135.3001) projected
  line L61 (0, 135.3001) -> (18.8297, 135.3001) projected
  line L62 (0, 135.3001) -> (0, 134.0127) projected
  line L63 (0, 134.0127) -> (-6, 116.3626) projected
  line L64 (-6, 116.3626) -> (-7.9242, 114.1104) projected
  line L65 (-7.9242, 114.1104) -> (-26.9242, 104.1104) projected
  line L66 (-26.9242, 104.1104) -> (-30.6501, 104.1104) projected
  line L67 (-30.6501, 104.1104) -> (-49.6501, 114.1104) projected
  line L68 (-49.6501, 114.1104) -> (-50.0258, 114.3352) projected
  line L69 (-50.0258, 114.3352) -> (-68.5062, 126.8156) projected
  line L70 (-68.5062, 126.8156) -> (-69.0444, 127.3537) projected
  line L71 (24.8297, 116.3626) -> (-6, 116.3626)
  circle A18 centre (9.4148, 116.3626) radius 14.5946
  circle A19 centre (-64.1166, 106.2401) radius 14.5946
  line L72 (-68.5062, 126.8156) -> (-50.0258, 114.3352) projected
  line L73 (-77.2122, 98.9398) -> (-81.0911, 112.5559) projected
  circle A20 centre (80.9704, 104.9058) radius 14.5946
  line L74 (100.068, 112.9805) -> (87.603, 82.65) projected
  line L75 (68.8555, 114.3352) -> (87.3359, 126.8156) projected
  line L76 (77.0633, 67.65) -> (-74.8673, 67.65)
  circle A21 centre (9.4148, 18.9375) radius 14.5946
  circle A22 centre (-64.1166, 29.06) radius 14.5946
  circle A23 centre (80.9704, 30.3943) radius 14.5946
  line L77 (-69.0444, 127.3537) -> (-82.4666, 113.9315) projected
  line L78 (-82.4666, 21.3686) -> (-69.0444, 7.9464) projected
  line L79 (101.1576, 114.0701) -> (87.874, 127.3537) projected
  line L80 (87.3359, 8.4845) -> (87.874, 7.9464) projected
  line L81 (87.874, 7.9464) -> (101.1576, 21.2299) projected
  point P0 (9.4148, 138.9501)
  point P1 (-78.1528, 102.2415)
  point P2 (-55.9486, 118.335)
  point P3 (-4.4032, 121.06)
  point P4 (23.2329, 121.06)
  point P5 (72.8024, 117.0006)
  point P6 (94.4695, 99.358)
  point P7 (94.4695, 35.9421)
  point P8 (72.8024, 18.2995)
  point P9 (-55.9486, 16.9651)
  point P10 (-78.1528, 33.0585)
  point P11 (23.2329, 14.2401)
  point P12 (-4.4032, 14.2401)
  dimension "d999" = 29.1892
  dimension "d1000" = 29.1892
  dimension "d1001" = 29.1892
  constraints: 6 centre point, 5 tangent, 4 end point, 3 midpoint, 3 symmetric about line, 1 horizontal, 3 other
  measures "d999" diameter of A19
  measures "d1000" diameter of A18
  measures "d1001" diameter of A20
extrude "Extrusion66" add sketch "Sketch71" along normal up to surface (45 mm away) contours L46 L45 L81 L80 L44 A23 | A20 L53 L52 L79 L51 L50 | L15 L14 L77 L70 L69 A19 | L28 L27 L78 L26 L25 A22 | L38 L37 L36 L35 L34 A21 | A18 L63 L62 L61 L60 L59
sketch "Sketch72" plane through (-13.202, -138.9501, 55) normal (0, -1, 0) x (1, 0, 0)
  line L0 (26.404, -45) -> (0, -45) projected
  line L1 (26.404, -45) -> (26.404, 0) projected
  line L2 (0, 0) -> (26.404, 0) projected
  line L3 (0, -45) -> (0, 0) projected
  circle A0 centre (13.202, -45) radius 27.3
  line L4 (0, 0) -> (26.404, 0)
  line L5 (26.404, 0) -> (26.404, -21.1045)
  line L6 (0, 0) -> (0, -21.1045)
  line L7 (13.202, 0) -> (13.202, -17.7)
  circle A1 centre (13.202, -45) radius 36.15
  line L8 (13.202, 0) -> (0, 0)
  line L9 (6.601, 0) -> (6.601, -18.5101)
  line L10 (19.803, 0) -> (19.803, -18.5101)
  line L11 (13.202, -17.7) -> (13.202, -8.85)
  circle A2 centre (13.202, -45) radius 31.725
  circle A3 centre (6.601, -13.9693) radius 2.5
  circle A4 centre (13.202, -13.275) radius 2.5
  circle A5 centre (19.803, -13.9693) radius 2.5
  point P0 (13.202, -55)
  dimension "d1005" = 72.3
  dimension "d1004" = 54.6
  dimension "d1006" = 63.45
  dimension "d1007" = 5
  dimension "d1008" = 5
  dimension "d1009" = 5
  constraints: 16 end point, 7 point on circle, 5 centre point, 5 midpoint, 4 point on line, 2 coincident, 2 collinear, 2 perpendicular, 2 symmetric about line, 1 vertical alignment, 2 other
  measures "d1004" diameter of A0
  measures "d1006" diameter of A2
  measures "d1007" diameter of A3
  measures "d1008" diameter of A4
  measures "d1009" diameter of A5
extrude "Extrusion67" cut sketch "Sketch72" against normal up to surface (135.3001 mm away) contours L0 L3 A0 L1 | A5 L10 A2 | A2 L10 A5 | A5 A2 L10 | A3 L9 A2 | A2 L9 A3 | L9 A2 A3 | A2 A5 L10 | A4 A2 L7 | L7 A2 A4 | L9 A3 A2 | A2 A4 L7 | L7 A4 A2 picked at (13.202, -35.9)
sketch "Sketch73" plane through (94.3529, -115.1101, 62.7835) normal (0.7071068, -0.7071068, 0) x (0.7071068, 0.7071068, 0)
  line L0 (0, -52.7835) -> (-26.404, -52.7835)
  line L1 (0, -52.7835) -> (0, -7.7835)
  line L2 (-26.404, -7.7835) -> (0, -7.7835)
  line L3 (-26.404, -52.7835) -> (-26.404, -7.7835)
  circle A0 centre (-13.202, -52.7835) radius 27.3
  line L4 (-26.404, -7.7835) -> (0, -7.7835)
  line L5 (0, -7.7835) -> (0, -28.8879)
  line L6 (-26.404, -7.7835) -> (-26.404, -28.8879)
  line L7 (-13.202, -7.7835) -> (-13.202, -25.4835)
  circle A1 centre (-13.202, -52.7835) radius 36.15
  line L8 (-13.202, -7.7835) -> (-26.404, -7.7835)
  line L9 (-19.803, -7.7835) -> (-19.803, -26.2936)
  line L10 (-6.601, -7.7835) -> (-6.601, -26.2936)
  line L11 (-13.202, -25.4835) -> (-13.202, -16.6335)
  circle A2 centre (-13.202, -52.7835) radius 31.725
  circle A3 centre (-19.803, -21.7528) radius 2.5
  circle A4 centre (-13.202, -21.0585) radius 2.5
  circle A5 centre (-6.601, -21.7528) radius 2.5
  line L12 (-26.404, -52.7835) -> (-26.404, -5.779) projected
  line L13 (0, -52.7835) -> (-26.404, -52.7835) projected
  line L14 (0, -52.7835) -> (0, 0) projected
  ellipse E0 centre (61.9567, -174.5872) end of major axis (316.5151, -174.5872) minor radius 180 (0, 0) -> (-26.404, -5.779) ccw projected
  point P0 (14.6775, -62.7835)
  point P1 (-13.202, -62.7835)
  dimension "d1013" = 72.3
  dimension "d1012" = 54.6
  dimension "d1014" = 63.45
  dimension "d1015" = 5
  dimension "d1016" = 5
  dimension "d1017" = 5
  dimension "d1018" = 90
  dimension "d1019" = 90
  dimension "d1020" = 90
  dimension "d1021" = 45
  dimension "d1022" = 6.601
  dimension "d1023" = 13.202
  dimension "d1024" = 121.8037
  dimension "d1025" = 10
  dimension "d1026" = 13.202
  constraints: 24 end point, 7 point on circle, 5 centre point, 5 midpoint, 4 point on line, 2 coincident, 2 collinear, 2 perpendicular, 2 symmetric about line, 1 horizontal, 1 vertical alignment, 3 other
  measures "d1012" diameter of A0
  measures "d1014" diameter of A2
  measures "d1015" diameter of A3
  measures "d1016" diameter of A4
  measures "d1017" diameter of A5
  measures "d1018" angle of L13 L5
  measures "d1019" angle of L14 L0
  measures "d1020" angle of L13 L6
  measures "d1021" distance between parallel lines of L13 L2
  measures "d1022" distance between parallel lines of L14 L10
  measures "d1023" distance between parallel lines of L14 L7
  measures "d1024" distance from line of point (61.957, -174.587) L0
  measures "d1025" distance from line of point (-13.202, -62.783) L13
  measures "d1026" distance from line of point (-13.202, -62.783) L14
extrude "Extrusion68" cut sketch "Sketch73" against normal blind 27 contours L0 L3 A0 L1 | A5 L10 A2 | A2 L10 A5 | A5 A2 L10 | A3 L9 A2 | A2 L9 A3 | L9 A2 A3 | A2 A5 L10 | A4 A2 L7 | L7 A2 A4 | L9 A3 A2 | A2 A4 L7 | L7 A4 A2 picked at (-13.202, -43.6835)
sketch "Sketch74" plane through (-94.3529, -115.1101, 62.7835) normal (-0.7071068, -0.7071068, 0) x (0.7071068, -0.7071068, 0)
  line L0 (26.404, -52.7835) -> (0, -52.7835)
  line L1 (26.404, -52.7835) -> (26.404, -7.7835)
  line L2 (0, -7.7835) -> (26.404, -7.7835)
  line L3 (0, -52.7835) -> (0, -7.7835)
  circle A0 centre (13.202, -52.7835) radius 27.3
  line L4 (0, -7.7835) -> (26.404, -7.7835)
  line L5 (26.404, -7.7835) -> (26.404, -28.8879)
  line L6 (0, -7.7835) -> (0, -28.8879)
  line L7 (13.202, -7.7835) -> (13.202, -25.4835)
  circle A1 centre (13.202, -52.7835) radius 36.15
  line L8 (13.202, -7.7835) -> (0, -7.7835)
  line L9 (6.601, -7.7835) -> (6.601, -26.2936)
  line L10 (19.803, -7.7835) -> (19.803, -26.2936)
  line L11 (13.202, -25.4835) -> (13.202, -16.6335)
  circle A2 centre (13.202, -52.7835) radius 31.725
  circle A3 centre (6.601, -21.7528) radius 2.5
  circle A4 centre (13.202, -21.0585) radius 2.5
  circle A5 centre (19.803, -21.7528) radius 2.5
  line L12 (26.404, -52.7835) -> (0, -52.7835) projected
  line L13 (26.404, -52.7835) -> (26.404, -5.779) projected
  ellipse E0 centre (-61.9567, -174.5872) end of major axis (-316.5151, -174.5872) minor radius 180 (26.404, -5.779) -> (0, 0) ccw projected
  line L14 (0, -52.7835) -> (0, 0) projected
  point P0 (-14.6775, -62.7835)
  point P1 (13.202, -62.7835)
  dimension "d1030" = 72.3
  dimension "d1029" = 54.6
  dimension "d1031" = 63.45
  dimension "d1032" = 5
  dimension "d1033" = 5
  dimension "d1034" = 5
  constraints: 24 end point, 7 point on circle, 5 centre point, 5 midpoint, 4 point on line, 2 coincident, 2 collinear, 2 perpendicular, 2 symmetric about line, 1 vertical alignment, 3 other
  measures "d1029" diameter of A0
  measures "d1031" diameter of A2
  measures "d1032" diameter of A3
  measures "d1033" diameter of A4
  measures "d1034" diameter of A5
extrude "Extrusion69" cut sketch "Sketch74" against normal blind 44 contours L0 L3 A0 L1 | A5 L10 A2 | A2 L10 A5 | A5 A2 L10 | A3 L9 A2 | A2 L9 A3 | L9 A2 A3 | A2 A5 L10 | A4 A2 L7 | L7 A2 A4 | L9 A3 A2 | A2 A4 L7 | L7 A4 A2 picked at (13.202, -43.6835)
sketch "Sketch75" plane through (-94.3529, -27.4901, 10) normal (-0.7071068, 0.7071068, 0) x (-0.7071068, -0.7071068, 0)
  line L0 (0, 0) -> (-26.404, 0)
  line L1 (0, 0) -> (0, 45)
  line L2 (-26.404, 45) -> (0, 45)
  line L3 (-26.404, 0) -> (-26.404, 45)
  circle A0 centre (-13.202, 0) radius 27.3
  line L4 (-26.404, 45) -> (0, 45)
  line L5 (0, 45) -> (0, 23.8955)
  line L6 (-26.404, 45) -> (-26.404, 23.8955)
  line L7 (-13.202, 45) -> (-13.202, 27.3)
  circle A1 centre (-13.202, 0) radius 36.15
  line L8 (-13.202, 45) -> (-26.404, 45)
  line L9 (-19.803, 45) -> (-19.803, 26.4899)
  line L10 (-6.601, 45) -> (-6.601, 26.4899)
  line L11 (-13.202, 27.3) -> (-13.202, 36.15)
  circle A2 centre (-13.202, 0) radius 31.725
  circle A3 centre (-19.803, 31.0307) radius 2.5
  circle A4 centre (-13.202, 31.725) radius 2.5
  circle A5 centre (-6.601, 31.0307) radius 2.5
  line L12 (-26.404, 0) -> (-26.404, 47.0045) projected
  line L13 (0, 0) -> (-26.404, 0) projected
  line L14 (0, 0) -> (0, 52.7835) projected
  ellipse E0 centre (61.9567, -121.8037) end of major axis (-192.6018, -121.8037) minor radius 180 (0, 52.7835) -> (-26.404, 47.0045) ccw projected
  point P0 (-86.156, -10)
  point P1 (-13.202, -10)
  dimension "d1038" = 72.3
  dimension "d1037" = 54.6
  dimension "d1039" = 63.45
  dimension "d1040" = 5
  dimension "d1041" = 5
  dimension "d1042" = 5
  constraints: 24 end point, 7 point on circle, 5 centre point, 5 midpoint, 4 point on line, 2 coincident, 2 collinear, 2 perpendicular, 2 symmetric about line, 1 vertical alignment, 3 other
  measures "d1037" diameter of A0
  measures "d1039" diameter of A2
  measures "d1040" diameter of A3
  measures "d1041" diameter of A4
  measures "d1042" diameter of A5
extrude "Extrusion70" cut sketch "Sketch75" against normal blind 44 contours L0 L3 A0 L1 | A5 L10 A2 | A2 L10 A5 | A5 A2 L10 | A3 L9 A2 | A2 L9 A3 | L9 A2 A3 | A2 A5 L10 | A4 A2 L7 | L7 A2 A4 | L9 A3 A2 | A2 A4 L7 | L7 A4 A2 picked at (-13.202, 9.1)
sketch "Sketch76" plane through (94.3529, -27.4901, 10) normal (0.7071068, 0.7071068, 0) x (-0.7071068, 0.7071068, 0)
  line L0 (26.404, 0) -> (0, 0)
  line L1 (26.404, 0) -> (26.404, 45)
  line L2 (0, 45) -> (26.404, 45)
  line L3 (0, 0) -> (0, 45)
  circle A0 centre (13.202, 0) radius 27.3
  line L4 (0, 45) -> (26.404, 45)
  line L5 (26.404, 45) -> (26.404, 23.8955)
  line L6 (0, 45) -> (0, 23.8955)
  line L7 (13.202, 45) -> (13.202, 27.3)
  circle A1 centre (13.202, 0) radius 36.15
  line L8 (13.202, 45) -> (0, 45)
  line L9 (6.601, 45) -> (6.601, 26.4899)
  line L10 (19.803, 45) -> (19.803, 26.4899)
  line L11 (13.202, 27.3) -> (13.202, 36.15)
  circle A2 centre (13.202, 0) radius 31.725
  circle A3 centre (6.601, 31.0307) radius 2.5
  circle A4 centre (13.202, 31.725) radius 2.5
  circle A5 centre (19.803, 31.0307) radius 2.5
  line L12 (26.404, 0) -> (0, 0) projected
  line L13 (26.404, 0) -> (26.404, 47.0045) projected
  ellipse E0 centre (-61.9567, -121.8037) end of major axis (192.6018, -121.8037) minor radius 180 (26.404, 47.0045) -> (0, 52.7835) ccw projected
  line L14 (0, 0) -> (0, 52.7835) projected
  point P0 (86.156, -10)
  point P1 (13.202, -10)
  dimension "d1046" = 72.3
  dimension "d1045" = 54.6
  dimension "d1047" = 63.45
  dimension "d1048" = 5
  dimension "d1049" = 5
  dimension "d1050" = 5
  constraints: 24 end point, 7 point on circle, 5 centre point, 5 midpoint, 4 point on line, 2 coincident, 2 collinear, 2 perpendicular, 2 symmetric about line, 1 vertical alignment, 3 other
  measures "d1045" diameter of A0
  measures "d1047" diameter of A2
  measures "d1048" diameter of A3
  measures "d1049" diameter of A4
  measures "d1050" diameter of A5
extrude "Extrusion71" cut sketch "Sketch76" against normal blind 44 contours L0 L3 A0 L1 | A5 L10 A2 | A2 L10 A5 | A5 A2 L10 | A3 L9 A2 | A2 L9 A3 | L9 A2 A3 | A2 A5 L10 | A4 A2 L7 | L7 A2 A4 | L9 A3 A2 | A2 A4 L7 | L7 A4 A2 picked at (13.202, 9.1)